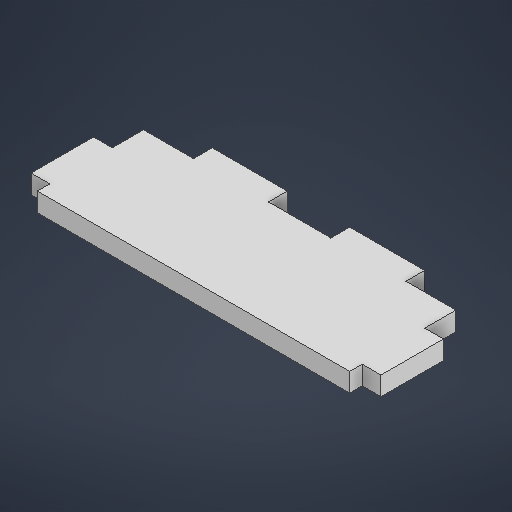
# Autodesk Inventor part: soporte_base_parqueo
Saved by Autodesk Inventor 2026 (Build 300175000, 175)
## iProperties
Created: 2026-05-15
Part Number: soporte_base_parqueo
Material: Generic
Document SubType Name: Modeling
Designer: juana
Density: 1 g/cm^3
Appearance: Default
Author: juana
Autodesk Inventor part; units mm, degrees
ref_plane "YZ Plane" through (0, 0, 0) normal (1, 0, 0) x (0, 1, 0)
ref_plane "XZ Plane" through (0, 0, 0) normal (0, 1, 0) x (-1, 0, 0)
ref_plane "XY Plane" through (0, 0, 0) normal (0, 0, 1) x (1, 0, 0)
sketch "Sketch1" plane through (0, 0, 0) normal (0, 1, 0) x (-1, 0, 0)
  line L0 (0, 0) -> (50, 0)
  line L1 (50, 0) -> (50, -20)
  line L2 (50, -20) -> (0, -20)
  line L3 (0, -20) -> (0, 0)
  line L4 (50, -2) -> (53, -2)
  line L5 (53, -2) -> (53, -12)
  line L6 (53, -12) -> (50, -12)
  line L7 (25, -20) -> (25, 0) construction
  line L8 (0, -2) -> (-3, -2)
  line L9 (-3, -2) -> (-3, -12)
  line L10 (-3, -12) -> (0, -12)
  line L11 (50, -17) -> (42, -17)
  line L12 (42, -17) -> (42, -20)
  line L13 (8, -20) -> (8, -17)
  line L14 (8, -17) -> (0, -17)
  line L15 (30, -17) -> (20, -17)
  line L16 (20, -17) -> (20, -20)
  line L17 (20, -20) -> (30, -20)
  line L18 (30, -20) -> (30, -17)
  point P0 (25, -17)
  point P1 (30, -20)
  dimension "d0" = 20
  dimension "d1" = 50
  dimension "d2" = 2
  dimension "d3" = 10
  dimension "d4" = 3
  dimension "d7" = 8
  dimension "d8" = 3
  dimension "d9" = 10
  constraints: 38 end point, 7 perpendicular, 7 point on line, 4 horizontal, 4 parallel, 4 symmetric about line, 3 midpoint, 2 horizontal alignment, 1 collinear, 1 vertical alignment
  measures "d0" distance of L0.end L1.end
  measures "d1" distance of L1.end L2.end
  measures "d2" distance between parallel lines of L0 L4
  measures "d3" distance of L4.end L5.end
  measures "d4" distance of L5.end L6.end
  measures "d7" distance of L11.start L11.end
  measures "d8" distance of L11.end L12.end
  measures "d9" distance of L15.start L15.end
extrude "Extrusion1" add sketch "Sketch1" along normal blind 3 contours L0 L1 L11 L12 L2 L18 L15 L16 L13 L14 L3 | L3 L10 L9 L8 | L4 L5 L6 L1
body "Solid1"
